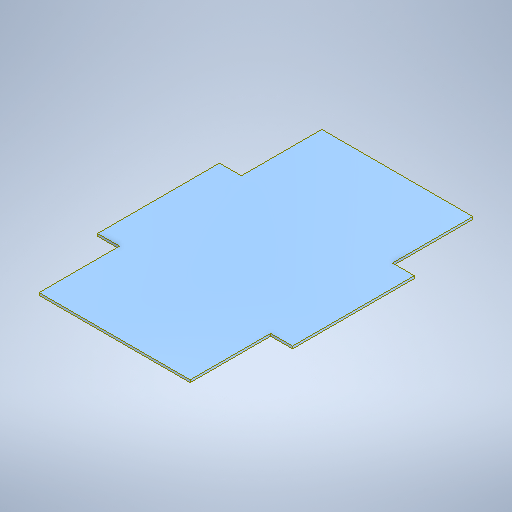
# Autodesk Inventor part: нижняя плита
Saved by Autodesk Inventor 2025 (Build 290162000, 162)
## iProperties
Created: 2025-01-21
Part Number: нижняя плита
Material: Типовые
Document SubType Name: Modeling
Designer: volko
Density: 1 g/cm^3
Appearance: По умолчанию
Author: volko
Autodesk Inventor part; units mm, degrees
ref_plane "YZ Plane" through (0, 0, 0) normal (1, 0, 0) x (0, 1, 0)
ref_plane "XZ Plane" through (0, 0, 0) normal (0, 1, 0) x (-1, 0, 0)
ref_plane "XY Plane" through (0, 0, 0) normal (0, 0, 1) x (1, 0, 0)
sketch "Эскиз1" plane through (0, 0, 0) normal (0, 1, 0) x (-1, 0, 0)
  line L0 (0, 290) -> (155, 290)
  line L1 (155, 290) -> (155, 125)
  line L2 (155, 125) -> (200, 125)
  line L3 (200, 125) -> (200, 0)
  line L4 (0, 290) -> (0, 0)
  line L5 (0, 0) -> (200, 0)
  line L6 (0, 290) -> (-155, 290)
  line L7 (-155, 290) -> (-155, 125)
  line L8 (-155, 125) -> (-200, 125)
  line L9 (-200, 125) -> (-200, 0)
  line L10 (0, -290) -> (155, -290)
  line L11 (155, -290) -> (155, -125)
  line L12 (155, -125) -> (200, -125)
  line L13 (200, -125) -> (200, 0)
  line L14 (-200, -125) -> (-200, 0)
  line L15 (-155, -125) -> (-200, -125)
  line L16 (-155, -290) -> (-155, -125)
  line L17 (0, -290) -> (-155, -290)
  point P0 (177.5, -125)
  point P1 (177.5, 125)
  dimension "d1" = 400
  dimension "d3" = 310
  dimension "d6" = 580
  dimension "d7" = 250
  constraints: 36 end point, 11 symmetric about line, 3 perpendicular, 2 midpoint, 2 point on line, 1 vertical
  measures "d1" distance between parallel lines of L9 L3
  measures "d3" distance between parallel lines of L7 L1
  measures "d6" distance between parallel lines of L6 L17
  measures "d7" distance of point (177.5, -125) point (177.5, 125)
extrude "Выдавливание1" add sketch "Эскиз1" along normal blind 5
